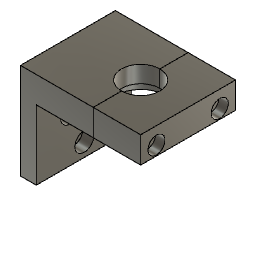
V6 MOUNT V1 v3 (Autodesk Fusion 360 design; units mm, degrees)
Autodesk Fusion 360 part; units mm, degrees
note: some values were not read from the file. Chosen so that the rebuilt part matches the saved one: which face or edge a step refers to.
sketch "Sketch1" plane through (0, 0, 0) normal (0, 0, 1) x (1, 0, 0)
  line L0 (15, -15) -> (-15, -15)
  line L1 (-15, -15) -> (-15, 15)
  line L2 (-15, 15) -> (15, 15)
  line L3 (15, 15) -> (15, -15)
  line L4 (15, -15) -> (-15, 15) construction
  line L5 (-15, -15) -> (15, 15) construction
  circle A0 centre (0, 0) radius 6.05
  line L6 (0, 0) -> (0, 15)
  line L7 (0, 0) -> (0, -15)
  dimension "d1" = 30
  dimension "d2" = 30
  dimension "d3" = 12.1
  constraint horizontal L0
  constraint perpendicular L0 L1
  constraint parallel L0 L2
  constraint parallel L1 L3
  constraint midpoint L2 L6.end
  constraint midpoint L0 L7.end
  measures "d1" distance of L1.end L2.end
  measures "d2" distance of L0.end L1.end
  measures "d3" diameter of A0
extrude "Extrude1" add sketch "Sketch1" along normal blind 6.1 contours L0 L2 L3 A0 L6 L7 makes body 1
extrude "Extrude2" add sketch "Sketch1" along normal blind 6.1 separate body contours L0 L1 L2 A0 L6 L7 makes body 2
sketch "Sketch2" plane through (15, 0, 0) normal (1, 0, 0) x (0, 1, 0)
  line L0 (-15, 0) -> (15, 0)
  line L1 (15, 0) -> (15, 6.1)
  line L2 (15, 6.1) -> (-15, 6.1)
  line L3 (-15, 6.1) -> (-15, 0)
  circle A0 centre (-10, 3) radius 1.52
  circle A1 centre (10, 3) radius 1.52
  dimension "d8" = 3.04
  dimension "d9" = 3.04
  measures "d8" diameter of A0
  measures "d9" diameter of A1
sketch "Sketch3" plane through (15, 0, 0) normal (1, 0, 0) x (0, 1, 0)
  circle A0 centre (-10, 3) radius 2.7
  circle A1 centre (10, 3) radius 2.7
  point P0 (-10, 3)
  point P1 (10, 3)
  dimension "d10" = 5.4
  dimension "d11" = 5.4
  constraint coincident P0 A0.centre
  constraint coincident P1 A1.centre
  measures "d10" diameter of A0
  measures "d11" diameter of A1
sketch "Sketch4" plane through (0, 0, 0) normal (0, 0, 1) x (1, 0, 0)
  circle A0 centre (0, 0) radius 8.05
  dimension "d12" = 16.1
  constraint coincident A0.centre origin
  measures "d12" diameter of A0
extrude "Extrude4" cut sketch "Sketch4" along normal blind 3 bodies 1 2
extrude "Extrude5" add 1 faces at (-12.011, -0.1507, 6.1) along direction (0, 0, 1) blind 3 on bodies 2 bodies 2
extrude "Extrude6" add 1 faces at (12.011, 0.1507, 6.1) along direction (0, 0, 1) blind 3 on bodies 1 bodies 1
extrude "Extrude7" cut sketch "Sketch2" against normal blind 30 contours A0 | A1 bodies 1 2
extrude "Extrude8" cut sketch "Sketch3" against normal blind 3 bodies 1
sketch "Sketch5" plane through (0, 0, 0) normal (1, 0, 0) x (0, 1, 0)
  line L0 (19.7, 13, -15) -> (16.7, 13, -15)
  line L1 (-15.3, 11.5, -15) -> (-15.3, 13, -15)
  line L2 (19.7, 11.5, -15) -> (14.7, 11.5, -15)
  circle A0 through (18.22, 13, -15) (15.94, 14.3164, -15) (15.94, 11.6836, -15)
  line L3 (20.8626, -30.5, -15) -> (20.8626, -29, -15)
  circle A1 through (12.7, -33.8977, -15) (-6.05, -23.0724, -15) (-6.05, -44.7231, -15)
  circle A2 through (-1.3013, -7.5859, -15) (-5.8013, -4.9878, -15) (-5.8013, -10.1839, -15)
  circle A3 through (-16.78, 13, -15) (-19.06, 14.3164, -15) (-19.06, 11.6836, -15)
  circle A4 through (6.2432, -7.5819, -15) (3.9632, -6.2655, -15) (3.9632, -8.8982, -15)
  circle A5 through (-15.8674, -29.0001, -15) (-18.1474, -27.6838, -15) (-18.1474, -30.3165, -15)
  line L4 (19.7, 11.5, -15) -> (19.7, 13, -15)
  circle A6 through (3.1987, -17.5859, -15) (-1.3013, -14.9878, -15) (-1.3013, -20.1839, -15)
  line L5 (20.8626, -29, -15) -> (17.6126, -29, -15)
  line L6 (-22.3, 21.1023, -15) -> (-22.3, -33.8977, -15)
  line L7 (-14.1374, -29.0001, -15) -> (-17.3874, -29.0001, -15)
  line L8 (22.7, 21.1023, -15) -> (-22.3, 21.1023, -15)
  circle A7 through (19.1326, -29, -15) (16.8526, -27.6836, -15) (16.8526, -30.3164, -15)
  circle A8 through (-2.7813, -7.5859, -15) (-5.0613, -6.2695, -15) (-5.0613, -8.9022, -15)
  circle A9 through (1.7187, -17.5859, -15) (-0.5613, -16.2695, -15) (-0.5613, -18.9022, -15)
  line L9 (-22.3, -33.8977, -15) -> (22.7, -33.8977, -15)
  line L10 (-15.3, 13, -15) -> (-18.3, 13, -15)
  line L11 (20.7301, -27.5039, -15) -> (14.2301, -27.5039, -15)
  line L12 (-13.8, -30.5, -15) -> (-13.8, -29, -15)
  line L13 (22.7, -33.8977, -15) -> (22.7, 21.1023, -15)
  circle A10 through (7.7232, -7.5819, -15) (3.2232, -4.9838, -15) (3.2232, -10.18, -15)
  dimension "d25" = 45
  dimension "d26" = 55
  dimension "d27" = 3.04
  dimension "d28" = 3.04
  dimension "d29" = 3.04
  dimension "d30" = 6
  dimension "d31" = 6
  dimension "d32" = 6
  dimension "d33" = 3.25
  dimension "d34" = 3.04
  dimension "d35" = 1.5
  dimension "d36" = 1.5
  dimension "d37" = 3.25
  dimension "d38" = 3.04
  dimension "d39" = 3
  dimension "d40" = 3.04
  dimension "d41" = 1.5
  dimension "d42" = 3
  dimension "d43" = 3.04
  dimension "d88" = 25
  dimension "d294" = 35
extrude "Extrude9" [suppressed]
sketch "Sketch6" plane through (-15, 0, 0) normal (1, 0, 0) x (0, 1, 0)
  line L0 (12.7, -33.8977) -> (22.7, -33.8977)
  line L1 (22.7, -33.8977) -> (22.7, 21.1023)
  line L2 (22.7, 21.1023) -> (-22.3, 21.1023)
  line L3 (-22.3, 21.1023) -> (-22.3, -33.8977)
  line L4 (-22.3, -33.8977) -> (-12.3, -33.8977)
  arc A0 (12.7, -33.8977) -> (-12.3, -33.8977) centre (0.2, -33.8977) ccw
  circle A1 centre (16.7, 13) radius 1.52
  circle A2 centre (-17.3874, -29.0001) radius 1.52
  circle A3 centre (17.6126, -29) radius 1.52
  circle A4 centre (-18.3, 13) radius 1.52
  line L5 (15, 0) -> (-15, 0)
  line L6 (-15, 0) -> (-15, 9.1)
  line L7 (-15, 9.1) -> (15, 9.1)
  line L8 (15, 9.1) -> (15, 0)
  line L9 (22.7, 21.1023) -> (20.2, 21.1023)
  line L10 (20.2, 21.1023) -> (20.2, 16.1023)
  line L11 (20.2, 16.1023) -> (22.7, 16.1023)
  line L12 (22.7, 16.1023) -> (22.7, 21.1023)
  line L13 (-22.3, 21.1023) -> (-19.8, 21.1023)
  line L14 (-19.8, 21.1023) -> (-19.8, 16.1023)
  line L15 (-19.8, 16.1023) -> (-22.3, 16.1023)
  line L16 (-22.3, 16.1023) -> (-22.3, 21.1023)
  dimension "d49" = 2.5
  dimension "d50" = 5
  dimension "d51" = 2.5
  dimension "d52" = 5
  constraint horizontal L9
  constraint vertical L10
  constraint horizontal L11
  constraint vertical L12
  constraint coincident L1.end L2.start
  constraint horizontal L13
  constraint vertical L14
  constraint horizontal L15
  constraint vertical L16
  constraint coincident L2.end L3.start
  measures "d49" distance of L1.end L9.end
  measures "d50" distance of L1.end L11.end
  measures "d51" distance of L2.end L13.end
  measures "d52" distance of L2.end L15.end
extrude "Extrude10" [suppressed]
sketch "Sketch7" plane through (0, 22.7, 0) normal (0, 1, 0) x (-1, 0, 0)
  line L0 (15, 16.1023) -> (15, -33.8977)
  line L1 (15, -33.8977) -> (20, -33.8977)
  line L2 (20, -33.8977) -> (20, 21.1023)
  line L3 (20, 21.1023) -> (7, 21.1023)
  line L4 (7, 21.1023) -> (7, 16.1023)
  line L5 (7, 16.1023) -> (15, 16.1023)
  circle A0 centre (11.7331, 18.6023) radius 1.5
  dimension "d55" = 3
  measures "d55" diameter of A0
extrude "Extrude11" [suppressed]
extrude "Extrude12" [suppressed]
sketch "Sketch8" plane through (-20, 0, 0) normal (-1, 0, 0) x (0, -1, 0)
  circle A0 centre (18.3, 13) radius 1.52
  circle A1 centre (-17.6126, -29) radius 1.52
  circle A2 centre (17.3874, -29.0001) radius 1.52
  circle A3 centre (-16.7, 13) radius 1.52
  line L0 (-22.7, -33.8977) -> (-12.7, -33.8977)
  arc A4 (12.3, -33.8977) -> (-12.7, -33.8977) centre (-0.2, -33.8977) ccw
  line L1 (12.3, -33.8977) -> (22.3, -33.8977)
  line L2 (22.3, -33.8977) -> (22.3, 21.1023)
  line L3 (22.3, 21.1023) -> (-22.7, 21.1023)
  line L4 (-22.7, 21.1023) -> (-22.7, -33.8977)
  circle A5 centre (-10, 3) radius 1.52
  circle A6 centre (10, 3) radius 1.52
  circle A7 centre (-10, 3) radius 2.7
  circle A8 centre (10, 3) radius 2.7
  dimension "d60" = 3.04
  dimension "d61" = 3.04
  dimension "d62" = 5.4
  dimension "d63" = 5.4
  constraint concentric A5 A7
  constraint concentric A6 A8
  measures "d60" diameter of A5
  measures "d61" diameter of A6
  measures "d62" diameter of A7
  measures "d63" diameter of A8
extrude "Extrude13" [suppressed]
extrude "Extrude14" [suppressed]
sketch "Sketch9" plane through (-15, 0, 0) normal (-1, 0, 0) x (0, -1, 0)
  circle A0 centre (-10, 3) radius 1.52
  circle A1 centre (10, 3) radius 1.52
  line L0 (-15, 0) -> (15, 0)
  line L1 (15, 0) -> (15, 9.1)
  line L2 (15, 9.1) -> (-15, 9.1)
  line L3 (-15, 9.1) -> (-15, 0)
  line L4 (-15, 9.1) -> (15, 9.1)
  line L5 (15, 9.1) -> (15, -22)
  line L6 (15, -22) -> (-15, -22)
  line L7 (-15, -22) -> (-15, 9.1)
  circle A2 centre (-4.7232, -7.5819) radius 1.52
  circle A3 centre (-4.7232, -7.5819) radius 3
  circle A4 centre (4.3013, -7.5859) radius 1.52
  circle A5 centre (4.3013, -7.5859) radius 3
  circle A6 centre (-0.1987, -17.5859) radius 1.52
  circle A7 centre (-0.1987, -17.5859) radius 3
  circle A8 centre (-10, 3) radius 2.7
  circle A9 centre (10, 3) radius 2.7
  point P0 (-4.7232, -7.5819)
  point P1 (4.3013, -7.5859)
  point P2 (-0.1987, -17.5859)
  dimension "d68" = 5.4
  dimension "d69" = 5.4
  constraint horizontal L4
  constraint vertical L5
  constraint horizontal L6
  constraint vertical L7
  constraint coincident L2.end L3.start
  constraint coincident P0 A2.centre
  constraint concentric A2 A3
  constraint coincident P1 A4.centre
  constraint coincident P2 A6.centre
  constraint concentric A0 A8
  constraint concentric A1 A9
  measures "d68" diameter of A8
  measures "d69" diameter of A9
extrude "Extrude15" add sketch "Sketch9" along normal blind 5 contours L0 L1 L2 L3 L4 L5 L7 | L0 L5 L6 L7 | A3 | A5 | A7 bodies 2
sketch "Sketch10" plane through (-20, 0, 0) normal (-1, 0, 0) x (0, -1, 0)
  circle A0 centre (10, 3) radius 2.7
  circle A1 centre (-10, 3) radius 2.7
  circle A2 centre (-0.1987, -17.5859) radius 1.52
  circle A3 centre (-4.7232, -7.5819) radius 1.52
  circle A4 centre (4.3013, -7.5859) radius 1.52
  line L0 (-15, -22) -> (15, -22)
  line L1 (15, -22) -> (15, 9.1)
  line L2 (15, 9.1) -> (-15, 9.1)
  line L3 (-15, 9.1) -> (-15, -22)
  circle A5 centre (-4.7232, -7.5819) radius 3
  circle A6 centre (4.3013, -7.5859) radius 3
  circle A7 centre (-0.1987, -17.5859) radius 3
  dimension "d72" = 6
  dimension "d73" = 6
  dimension "d74" = 6
  constraint concentric A3 A5
  constraint concentric A4 A6
  constraint concentric A2 A7
  measures "d72" diameter of A7
  measures "d73" diameter of A6
  measures "d74" diameter of A5
extrude "Extrude16" cut sketch "Sketch9" along normal blind 3.2 contours A3 | A5 | A7 bodies 2
sketch "Sketch11" plane through (0, 0, 9.1) normal (0, 0, 1) x (-1, 0, 0)
  line L0 (0, -6.05) -> (0, -15)
  line L1 (0, -15) -> (20, -15)
  line L2 (20, -15) -> (20, 15)
  line L3 (20, 15) -> (0, 15)
  line L4 (0, 15) -> (0, 6.05)
  arc A0 (0, -6.05) -> (0, 6.05) centre (0, 0) ccw
extrude "Extrude17" add sketch "Sketch10" along normal blind 3 contours L0 L1 L2 L3 | A5 | A6 | A7 bodies 2
extrude "Extrude18" cut sketch "Sketch9" along normal blind 3 contours L0 L5 L6 L7 bodies 2
extrude "Extrude19" cut sketch "Sketch9" along normal blind 6.5 contours A3 | A5 | A7 bodies 2
extrude "Extrude20" cut 1 faces at (-16.3444, 0.1507, 9.1) along direction (0, 0, -1) blind 0.8 on bodies 2 bodies 2
extrude "Extrude21" cut 1 faces at (12.011, 0.1507, 9.1) along direction (0, 0, -1) blind 0.8 on bodies 1 bodies 1
